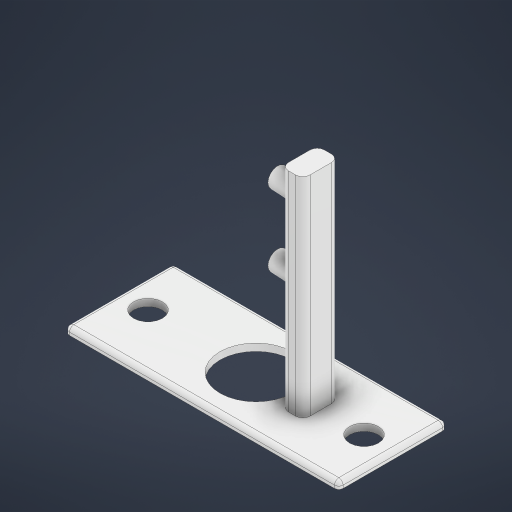
# Autodesk Inventor part: sensor_holder
Saved by Autodesk Inventor 2024.4 (Build 284460000, 460)
## iProperties
Created: 2026-02-14
Part Number: sensor_holder
Material: Tworzywo sztuczne ABS
Document SubType Name: Modeling
Designer: User
Density: 1.06 g/cm^3
Appearance: Gładki — biały
Author: User
Autodesk Inventor part; units mm, degrees
ref_plane "YZ Plane" through (0, 0, 0) normal (1, 0, 0) x (0, 1, 0)
ref_plane "XZ Plane" through (0, 0, 0) normal (0, 1, 0) x (-1, 0, 0)
ref_plane "XY Plane" through (0, 0, 0) normal (0, 0, 1) x (1, 0, 0)
sketch "Szkic1" plane through (0, 0, 0) normal (0, 1, 0) x (-1, 0, 0)
  line L0 (0, 0) -> (-15, 0)
  line L1 (0, 0) -> (15, 0)
  circle A0 centre (0, 0) radius 5
  circle A1 centre (15, 0) radius 2
  circle A2 centre (-15, 0) radius 2
  line L2 (-19, 7.5) -> (19, 7.5)
  line L3 (19, 7.5) -> (19, -7.5)
  line L4 (19, -7.5) -> (-19, -7.5)
  line L5 (-19, -7.5) -> (-19, 7.5)
  line L6 (-19, 7.5) -> (19, -7.5) construction
  line L7 (19, 7.5) -> (-19, -7.5) construction
  line L8 (0, 0) -> (15, 0)
  line L9 (6, 2.5) -> (9, 2.5)
  line L10 (9, 2.5) -> (9, -2.5)
  line L11 (9, -2.5) -> (6, -2.5)
  line L12 (6, -2.5) -> (6, 2.5)
  line L13 (6, 2.5) -> (9, -2.5) construction
  line L14 (9, 2.5) -> (6, -2.5) construction
  line L15 (-9, 2.5) -> (-6, 2.5)
  line L16 (-6, 2.5) -> (-6, -2.5)
  line L17 (-6, -2.5) -> (-9, -2.5)
  line L18 (-9, -2.5) -> (-9, 2.5)
  line L19 (-9, 2.5) -> (-6, -2.5) construction
  line L20 (-6, 2.5) -> (-9, -2.5) construction
  point P0 (7.5, 0)
  point P1 (-7.5, 0)
  point P2 (-5, 0)
  point P3 (5, 0)
  dimension "d0" = 15
  dimension "d1" = 15
  dimension "d2" = 10
  dimension "d3" = 4
  dimension "d4" = 4
  dimension "d5" = 38
  dimension "d6" = 15
  dimension "d7" = 3
  dimension "d8" = 5
  dimension "d9" = 3
  dimension "d10" = 5
  constraints: 42 end point, 8 midpoint, 6 horizontal, 6 parallel, 3 centre point, 3 coincident, 3 perpendicular
  measures "d0" distance of L0.start L0.end
  measures "d1" distance of L0.start L1.end
  measures "d2" diameter of A0
  measures "d3" diameter of A1
  measures "d4" diameter of A2
  measures "d5" distance of L3.end L4.end
  measures "d6" distance of L2.end L3.end
  measures "d7" distance of L10.end L11.end
  measures "d8" distance of L9.end L10.end
  measures "d9" distance of L16.end L17.end
  measures "d10" distance of L15.end L16.end
extrude "Wyciągnięcie proste1" add sketch "Szkic1" along normal blind 1 contours L16 L17 L18 L0 | L0 L18 L15 L16 | L12 L9 L10 L1 | L1 L10 L11 L12 | L2 L3 L4 L5
extrude "Wyciągnięcie proste2" add sketch "Szkic1" along normal blind 30 contours L16 L17 L18 L0 | L0 L18 L15 L16
sketch "Szkic2" plane through (-6, 1, -2.5) normal (1, 0, 0) x (0, 0, -1)
  line L0 (0, 19) -> (-5, 19)
  line L1 (0, 19) -> (-2.12132, 16.87868)
  line L2 (0, 19) -> (3, 19) construction
  circle A0 centre (-2.12132, 16.87868) radius 1.5
  point P0 (-2.5, -1)
  dimension "d15" = 3
  dimension "d16" = 135
  dimension "d17" = 3
  constraints: 4 end point, 1 centre point, 1 coincident, 1 equal length, 1 horizontal
  measures "d15" distance of L0.start L1.end
  measures "d16" angle of L1 L2
  measures "d17" diameter of A0
extrude "Wyciągnięcie proste3" [suppressed]
fillet "Zaokrąglenie1" radius 1 4 edges at (6, 15.5, -2.5) (9, 15.5, -2.5) (9, 15.5, 2.5) (6, 15.5, 2.5)
sketch "Szkic3" plane through (6, 1, 1.5) normal (-1, 0, 0) x (0, 0, 1)
  line L0 (-1.5, 27) -> (-1.5, 25)
  circle A0 centre (-1.5, 25) radius 1.5
  line L1 (-1.5, 25) -> (-1.5, 15)
  circle A1 centre (-1.5, 15) radius 1.5
  line L2 (-3, 29) -> (0, 29) projected
  point P0 (-1.5, -1)
  point P1 (0, 19)
  point P2 (-3, 19)
  point P3 (-1.5, 29)
  dimension "d21" = 2
  dimension "d22" = 3
  dimension "d23" = 10
  dimension "d24" = 3
  dimension "d28" = 2
  constraints: 4 end point, 2 centre point, 2 coincident, 2 vertical, 1 midpoint
  measures "d21" distance of L0.start L0.end
  measures "d22" diameter of A0
  measures "d23" distance of L1.start L1.end
  measures "d24" diameter of A1
  measures "d28" distance of point (-1.5, 29) L0.start
sketch "Szkic3 outline for Wyciągnięcie proste4" plane through (6, 1, 1.5) normal (-1, 0, 0) x (0, 0, 1)
  circle A0 centre (-1.5, 25) radius 1.5
  circle A1 centre (-1.5, 15) radius 1.5
extrude "Wyciągnięcie proste4" add sketch "Szkic3 outline for Wyciągnięcie proste4" along normal blind 3 draft -3
fillet "Zaokrąglenie2" radius 0.6 8 edges at (-19, 0.5, 7.5) (-19, 0.5, -7.5) (-19, 1, 0) (0, 1, 7.5) (19, 1, 0) (19, 0.5, 7.5) (19, 0.5, -7.5) (0, 1, -7.5)
